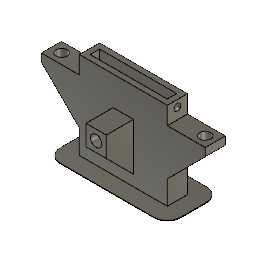
smmb_coin-thrower (Autodesk Fusion 360 design; units mm, degrees)
Autodesk Fusion 360 part; units mm, degrees
note: some values were not read from the file. Set by a fixed rule: which sketch regions a step uses.
sketch "Sketch1" plane through (0, 0, 0) normal (0, 0, 1) x (1, 0, 0)
  line L0 (0, 0) -> (28.5, 0)
  line L1 (28.5, 0) -> (28.5, 3.5)
  line L2 (28.5, 3.5) -> (0, 3.5)
  line L3 (0, 3.5) -> (0, 0)
  line L4 (-2, -2) -> (30.5, -2)
  line L5 (30.5, -2) -> (30.5, 5.5)
  line L6 (30.5, 5.5) -> (-2, 5.5)
  line L7 (-2, 5.5) -> (-2, -2)
  line L8 (-3, -8) -> (31.5, -8)
  line L9 (36.5, -3) -> (36.5, 6.5)
  line L10 (31.5, 11.5) -> (-3, 11.5)
  line L11 (-8, 6.5) -> (-8, -3)
  arc A0 (-3, 11.5) -> (-8, 6.5) centre (-3, 6.5) ccw
  arc A1 (36.5, 6.5) -> (31.5, 11.5) centre (31.5, 6.5) ccw
  arc A2 (31.5, -8) -> (36.5, -3) centre (31.5, -3) ccw
  arc A3 (-8, -3) -> (-3, -8) centre (-3, -3) ccw
  dimension "d1" = 28.5
  dimension "d2" = 3.5
  dimension "d3" = 2
  dimension "d48" = 5
  constraint horizontal L0
  constraint vertical L1
  constraint horizontal L2
  constraint vertical L3
  constraint coincident L0.start L3.end
  constraint parallel L0 L8
  constraint parallel L1 L9
  constraint parallel L2 L10
  constraint parallel L3 L11
  constraint tangent L11 A0
  constraint tangent L10 A0
  constraint tangent L10 A1
  constraint tangent L9 A1
  constraint equal A0 A1
  constraint tangent L9 A2
  constraint tangent L8 A2
  constraint equal A0 A2
  constraint tangent L8 A3
  constraint tangent L11 A3
  constraint equal A0 A3
  measures "d1" distance of L0.start L0.end
  measures "d2" distance of L0.start L2.end
  measures "d48" radius of A0
extrude "Extrude1" add sketch "Sketch1" along normal blind 32.5 contours L4 L5 L6 L7
ref_plane "WorkPlane3" through (14.25, 1.75, 26) normal (0, 0, 1) x (1, 0, 0)
sketch "Sketch5" plane through (0, -2, 0) normal (0, -1, 0) x (1, 0, 0)
  line L0 (-2, 0) -> (30.5, 0)
  line L1 (30.5, 0) -> (30.5, 32.5)
  line L2 (30.5, 32.5) -> (-2, 32.5)
  line L3 (-2, 32.5) -> (-2, 0)
  line L4 (-5.25, 26) -> (33.75, 26)
  circle A0 centre (14.25, 18) radius 2.1
  line L5 (18, 21.75) -> (10.5, 21.75)
  line L6 (10.5, 21.75) -> (10.5, 14.25)
  line L7 (10.5, 14.25) -> (18, 14.25)
  line L8 (18, 14.25) -> (18, 21.75)
  line L9 (18, 21.75) -> (10.5, 14.25) construction
  line L10 (10.5, 21.75) -> (18, 14.25) construction
  line L11 (-2, 0) -> (30.5, 0)
  point P0 (14.25, 18)
  dimension "d27" = 4.2
  dimension "d28" = 7.5
  dimension "d29" = 7.5
  dimension "d30" = 8
  constraint perpendicular L5 L6
  constraint parallel L5 L7
  constraint parallel L6 L8
  constraint horizontal L5
  constraint coincident L9 P0
  constraint coincident L10 P0
  constraint coincident P0 A0.centre
  measures "d27" diameter of A0
  measures "d28" distance of L5.end L6.end
  measures "d29" distance of L6.end L7.end
  measures "d30" distance of L4 P0
extrude "Extrude3" add sketch "Sketch5" along normal blind 10 contours L5 L6 L7 L8
sketch "Sketch6" plane through (30.5, 0, 0) normal (1, 0, 0) x (0, 1, 0)
  line L0 (-2, 0) -> (5.5, 0)
  line L1 (5.5, 0) -> (5.5, 32.5)
  line L2 (5.5, 32.5) -> (-2, 32.5)
  line L3 (-2, 32.5) -> (-2, 0)
  line L4 (6.25, 26) -> (-2.75, 26)
  circle A0 centre (1.75, 30) radius 1.25
  line L5 (1.75, 31.25) -> (1.75, 28.75)
  dimension "d36" = 2.5
  dimension "d37" = 3.75
  dimension "d38" = 2.5
  dimension "d39" = 2.5
  constraint coincident A0 L5.start
  constraint coincident A0 L5.end
  constraint vertical L5
  measures "d36" diameter of A0
  measures "d37" distance of L3 A0.centre
  measures "d38" distance of L2 A0.centre
  measures "d39" distance of L5.start L5.end
revolve "Revolve1" cut sketch "Sketch6" angle 360 about axis through (30.5, 1.75, 31.25) along (0, 0, -1) contours A0 L5 picked at (2.4551, 29.6422)
sketch "Sketch7" plane through (-2, 0, 0) normal (-1, 0, 0) x (0, -1, 0)
  line L0 (-5.5, 0) -> (2, 0)
  line L1 (2, 0) -> (2, 32.5)
  line L2 (2, 32.5) -> (-5.5, 32.5)
  line L3 (-5.5, 32.5) -> (-5.5, 0)
  line L4 (-6.25, 26) -> (2.75, 26)
  circle A0 centre (-1.75, 30) radius 1.25
  line L5 (-1.75, 31.25) -> (-1.75, 28.75)
  point P0 (-1.75, 31.25)
  dimension "d41" = 2.5
  dimension "d42" = 3.75
  dimension "d43" = 2.5
  constraint coincident P0 L5.start
  constraint coincident A0 L5.end
  constraint vertical L5
  measures "d41" diameter of A0
  measures "d42" distance of L3 A0.centre
  measures "d43" distance of L2 A0.centre
revolve "Revolve2" cut sketch "Sketch7" angle 360 about axis through (-2, 1.75, 31.25) along (0, 0, -1) contours A0 L5 picked at (-1.2448, 29.6517)
extrude "Extrude4" add sketch "Sketch1" along normal blind 0.25 contours L8 L9 L10 L11 A0 A1 A2 A3
sketch "Sketch8" plane through (14.25, 1.75, 26) normal (0, 0, 1) x (1, 0, 0)
  line L0 (16.25, -3.75) -> (16.25, 3.75)
  line L1 (16.25, -3.75) -> (30.25, -3.75)
  line L2 (30.25, -3.75) -> (30.25, 3.75)
  line L3 (30.25, 3.75) -> (16.25, 3.75)
  line L4 (16.25, 3.75) -> (16.25, -3.75)
  circle A0 centre (26.5, 0) radius 2.05
  circle A1 centre (26.5, 0) radius 3.55
  line L5 (-14.25, -1.75) -> (14.25, -1.75)
  line L6 (14.25, 1.75) -> (-14.25, 1.75)
  line L7 (0, -1.75) -> (0, 1.75)
  line L8 (-16.25, -3.75) -> (-16.25, 3.75)
  line L9 (-16.25, 3.75) -> (-16.25, -3.75)
  line L10 (-16.25, -3.75) -> (-30.25, -3.75)
  line L11 (-30.25, -3.75) -> (-30.25, 3.75)
  circle A2 centre (-26.5, 0) radius 2.05
  line L12 (-30.25, 3.75) -> (-16.25, 3.75)
  circle A3 centre (-26.5, 0) radius 3.55
  dimension "d51" = 7.5
  dimension "d52" = 14
  dimension "d53" = 4.1
  dimension "d54" = 3.75
  dimension "d55" = 3.75
  dimension "d56" = 7.1
  constraint horizontal L1
  constraint vertical L2
  constraint horizontal L3
  constraint vertical L4
  constraint coincident L0.start L1.start
  constraint concentric A0 A1
  constraint midpoint L5 L7.start
  constraint midpoint L6 L7.end
  constraint symmetric L0.start L7 L8.start
  constraint symmetric L0.end L7 L8.end
  constraint symmetric L1.end L7 L10.end
  constraint symmetric L2.end L7 L11.end
  constraint symmetric A0 L7 A2
  constraint symmetric A1 L7 A3
  measures "d51" distance of L0.start L0.end
  measures "d52" distance of L0.start L1.end
  measures "d53" diameter of A0
  measures "d54" distance of L3 A0.centre
  measures "d55" distance of L2 A0.centre
  measures "d56" diameter of A1
extrude "Extrude6" add sketch "Sketch8" against normal blind 3 contours L0 L1 L2 L3 L4 | A0 | A1 | L8 L9 L10 L11 L12 | A2 | A3
chamfer "Chamfer3" distance 10 distance2 10 1 edges at (14.25, -2, 14.25) measured on face at (13, -2, 4.9167)
chamfer "Chamfer4" distance 14 angle 45 2 edges at (-2, 1.75, 23) (30.5, 1.75, 23)
extrude "Extrude7" cut sketch "Sketch8" against normal blind 4 contours A0 | A2
equation "d6 = 26 mm + 1.5 mm + 5 mm"
equation "d39 = d36"
equation "d54 = d51 / 2"
equation "d55 = d54"
equation "d56 = d53 + 3 mm"
